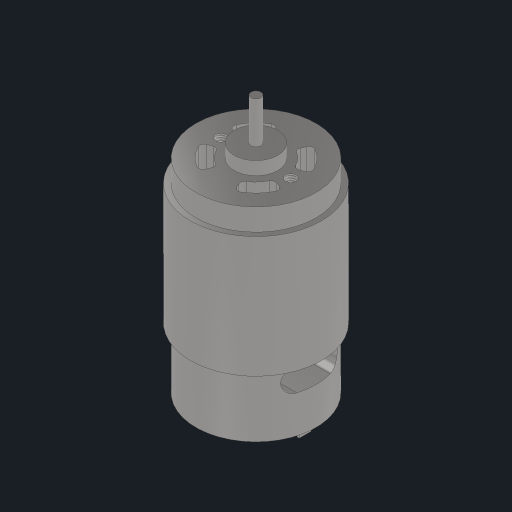
# Autodesk Inventor part: rs390
Saved by Autodesk Inventor 2023 (Build 270158000, 158)
## iProperties
Created: 2024-04-13
Part Number: rs390
Material: Steel, Mild
Document SubType Name: Modeling
Designer: szymo
Density: 3.97435 g/cm^3
Appearance: Semi-Polished
Mass: 115 g
Surface Area: 75.062 cm^2
Volume: 28.9356 cm^3
Author: szymo
Autodesk Inventor part; units mm, degrees
ref_plane "YZ Plane" through (0, 0, 0) normal (1, 0, 0) x (0, 1, 0)
sketch "Sketch1" plane through (0, 0, 0) normal (0, 1, 0) x (-1, 0, 0)
  circle A0 centre (0, 0) radius 13.75
  dimension "d0" = 27.5
  constraints: 1 centre point, 1 coincident
  measures "d0" diameter of A0
extrude "Extrusion1" add sketch "Sketch1" along normal blind 46.6
sketch "Sketch2" plane through (0, 46.6, 0) normal (0, 1, 0) x (1, 0, 0)
  circle A0 centre (0, 0) radius 13.75 projected
  circle A1 centre (0, 0) radius 5
  dimension "d3" = 10
  constraints: 1 centre point, 1 coincident
  measures "d3" diameter of A1
extrude "Extrusion2" add sketch "Sketch2" along normal blind 3 contours A1
sketch "Sketch3" plane through (0, 46.6, 0) normal (0, 1, 0) x (1, 0, 0)
  circle A0 centre (0, 0) radius 5 projected
  circle A1 centre (0, 0) radius 5 projected
  circle A2 centre (0, 0) radius 13.75 projected
  circle A3 centre (0, 0) radius 13.75 projected
  line L0 (-13.75, 0) -> (13.75, 0)
  point P0 (-8, 0)
  point P1 (8, 0)
  dimension "d6" = 16
  dimension "d7" = 5.75
  dimension "d8" = 5.75
  constraints: 2 end point, 2 point on circle, 2 point on line, 1 horizontal, 1 midpoint
  measures "d6" distance of point (-8, 0) point (8, 0)
  measures "d7" distance of L0.start point (-8, 0)
  measures "d8" distance of L0.end point (8, 0)
hole "Hole1" at (-8, 46.6, 0) at (8, 46.6, 0) direction (0, -1, 0) diameter 2.459 depth 3 thread size "M3x0.5" class "6H" standard "ISO Metric profile"
ref_plane "Work Plane1" through (0, 41.6, 0) normal (0, 1, 0) x (1, 0, 0)
sketch "Sketch4" plane through (0, 41.6, 0) normal (0, 1, 0) x (1, 0, 0)
  circle A0 centre (0, 0) radius 15
  dimension "d17" = 30
  constraints: 1 centre point, 1 coincident
  measures "d17" diameter of A0
extrude "Extrusion3" add sketch "Sketch4" against normal blind 27.7
sketch "Sketch5" plane through (0, 0, 0) normal (0, -1, 0) x (1, 0, 0)
  circle A0 centre (0, 0) radius 5
  dimension "d20" = 10
  constraints: 1 centre point, 1 coincident
  measures "d20" diameter of A0
extrude "Extrusion4" add sketch "Sketch5" along normal blind 2.7
sketch "Sketch6" plane through (0, 0, 0) normal (0, -1, 0) x (1, 0, 0)
  circle A0 centre (0, 0) radius 5 projected
  circle A1 centre (0, 0) radius 5 projected
  circle A2 centre (0, 0) radius 13.75 projected
  circle A3 centre (0, 0) radius 13.75 projected
  line L0 (13.75, 0) -> (-13.75, 0)
  line L1 (-11.25, 1.35) -> (-11.75, 1.35)
  line L2 (-11.75, 1.35) -> (-11.75, -1.35)
  line L3 (-11.75, -1.35) -> (-11.25, -1.35)
  line L4 (-11.25, -1.35) -> (-11.25, 1.35)
  line L5 (11.25, 1.35) -> (10.75, 1.35)
  line L6 (10.75, 1.35) -> (10.75, -1.35)
  line L7 (10.75, -1.35) -> (11.25, -1.35)
  line L8 (11.25, -1.35) -> (11.25, 1.35)
  dimension "d23" = 22
  dimension "d24" = 0.5
  dimension "d25" = 0.5
  dimension "d26" = 11.25
  dimension "d27" = 11.25
  dimension "d28" = 2.7
  dimension "d29" = 2.7
  dimension "d30" = 1.35
  dimension "d31" = 1.35
  constraints: 18 end point, 4 horizontal, 4 parallel, 2 perpendicular, 2 point on circle, 2 point on line
  measures "d23" distance between parallel lines of L6 L4
  measures "d24" distance of L6.end L7.end
  measures "d25" distance between parallel lines of L4 L2
  measures "d26" distance from line of A2.centre L8
  measures "d27" distance from line of A0.centre L4
  measures "d28" distance between parallel lines of L3 L1
  measures "d29" distance of L7.end L5.start
  measures "d30" distance between parallel lines of L0 L7
  measures "d31" distance between parallel lines of L0 L5
extrude "Extrusion5" add sketch "Sketch6" along normal up to surface (2.7 mm away) contours L6 L5 L8 L0 | L0 L8 L7 L6 | L4 L3 L2 L0 | L0 L2 L1 L4
sketch "Sketch7" plane through (0, 49.6, 0) normal (0, 1, 0) x (1, 0, 0)
  circle A0 centre (0, 0) radius 1.15
  dimension "d34" = 2.3
  constraints: 1 centre point, 1 coincident
  measures "d34" diameter of A0
extrude "Extrusion6" add sketch "Sketch7" along normal blind 9.5
ref_plane "Work Plane2" through (0, 50.6, 0) normal (0, 1, 0) x (1, 0, 0)
sketch "Sketch10" plane through (0, 0, 0) normal (1, 0, 0) x (0, 1, 0)
  line L0 (0, -13.75) -> (0, 13.75) projected
  line L1 (13.9, 13.75) -> (13.9, -13.75) projected
  line L2 (8.5, 3.8) -> (13.9, 3.8)
  line L3 (13.9, 3.8) -> (13.9, -3.8)
  line L4 (13.9, -3.8) -> (8.5, -3.8)
  line L5 (8.5, -3.8) -> (8.5, 3.8)
  circle A0 centre (11.2, 3.8) radius 2.7
  circle A1 centre (11.2, -3.8) radius 2.7
  line L6 (0, 0) -> (13.9, 0)
  line L7 (13.9, 13.75) -> (13.9, -13.75) projected
  line L8 (0, -13.75) -> (13.9, -13.75) projected
  point P0 (11.2, -6.5)
  point P1 (11.2, 6.5)
  dimension "d57" = 8.5
  dimension "d59" = 0
  dimension "d60" = 5.4
  dimension "d61" = 13.9
  dimension "d65" = 3.8
  dimension "d66" = 3.8
  dimension "d80" = 5.4
  dimension "d81" = 5.4
  dimension "d82" = 2.7
  dimension "d83" = 2.7
  dimension "d84" = 13
  constraints: 10 end point, 4 point on circle, 3 midpoint, 2 centre point, 2 parallel, 1 horizontal, 1 perpendicular
  measures "d57" distance between parallel lines of L0 L5
  measures "d59" distance between parallel lines of L3 L1
  measures "d60" distance between parallel lines of L5 L1
  measures "d61" distance between parallel lines of L0 L1
  measures "d65" distance from line of L6 A0.centre
  measures "d66" distance from line of L6 A1.centre
  measures "d80" diameter of A1
  measures "d81" diameter of A0
  measures "d82" distance from line of L1 A1.end
  measures "d83" distance from line of L1 A0.end
  measures "d84" distance of A0.end A1.end
extrude "Extrusion9" cut sketch "Sketch10" along normal mid plane 31.5 contours L6 L1 A1 L5 | L5 A0 L1 L6 | A1 L4 | L4 A1 | A0 L2 | L2 A0
sketch "Sketch12" plane through (0, 46.6, 0) normal (0, 1, 0) x (1, 0, 0)
  circle A0 centre (0, 0) radius 1.15 projected
  circle A1 centre (0, 0) radius 5 projected
  circle A2 centre (-8, 0) radius 1.2295 projected
  circle A3 centre (8, 0) radius 1.2295 projected
  circle A4 centre (0, 0) radius 5 projected
  circle A5 centre (0, 0) radius 13.75 projected
  circle A6 centre (0, 0) radius 13.75 projected
  line L0 (-13.75, 0) -> (13.75, 0)
  line L1 (0, 13.75) -> (0, -13.75)
  circle A7 centre (0, 0) radius 6.7705
  circle A8 centre (0, 0) radius 9.8705
  line L2 (-2.75, 6.1869) -> (-4.0091, 9.0196)
  line L3 (-6.3854, 2.2508) -> (-9.3091, 3.2814)
  line L4 (2.75, 6.1869) -> (4.0091, 9.0196)
  line L5 (6.3854, 2.2508) -> (9.3091, 3.2814)
  circle A9 centre (-8, 0) radius 1.2295 projected
  circle A10 centre (8, 0) radius 1.2295 projected
  line L6 (-2.75, -6.1869) -> (-4.0091, -9.0196)
  line L7 (-6.3854, -2.2508) -> (-9.3091, -3.2814)
  line L8 (2.75, -6.1869) -> (4.0091, -9.0196)
  line L9 (6.3854, -2.2508) -> (9.3091, -3.2814)
  point P0 (0, 6.7705)
  point P1 (0, 9.8705)
  point P2 (-8, 1.2295)
  point P3 (8, 1.2295)
  dimension "d85" = 3.1
  dimension "d86" = 5.5
  dimension "d87" = 4.0091
  dimension "d88" = 4.0091
  dimension "d89" = 1.5
  dimension "d90" = 1.5
  dimension "d91" = 1.2295
  dimension "d92" = 2.459
  dimension "d93" = 2.459
  dimension "d94" = 1.2295
  constraints: 20 end point, 14 point on circle, 8 symmetric about line, 4 line through centre, 3 midpoint, 2 centre point, 2 coincident, 2 point on line, 2 vertical alignment, 1 horizontal, 1 tangent, 1 vertical, 2 other
  measures "d85" distance of A7.start A8.start
  measures "d86" distance of L4.start L2.start
  measures "d87" distance from line of L1 L4.end
  measures "d88" horizontal distance of L2.end A8.start
  measures "d89" distance from line of point (-8, 1.23) L3
  measures "d90" distance from line of L5 point (8, 1.23)
  measures "d91" distance from line of L0 point (-8, 1.23)
  measures "d92" diameter of A2
  measures "d93" diameter of A3
  measures "d94" distance of A3.centre point (8, 1.23)
extrude "Extrusion11" cut sketch "Sketch12" against normal blind 10 contours A7 L4 A8 L5 | L9 A8 L8 A7 | A7 L3 A8 L2 | L6 A8 L7 A7
fillet "Fillet1" radius 1 16 edges at (-4.0091, 41.6, -9.0196) (-2.75, 41.6, -6.1869) (-6.3854, 41.6, -2.2508) (-9.3091, 41.6, -3.2814) (9.3091, 41.6, -3.2814) (6.3854, 41.6, -2.2508) (4.0091, 41.6, -9.0196) (9.3091, 41.6, 3.2814) (6.3854, 41.6, 2.2508) (4.0091, 41.6, 9.0196) (2.75, 41.6, 6.1869) (-4.0091, 41.6, 9.0196) (-9.3091, 41.6, 3.2814) (-6.3854, 41.6, 2.2508) (-2.75, 41.6, 6.1869) (2.75, 41.6, -6.1869)
sketch "Sketch13" plane through (0, -2.7, 0) normal (0, -1, 0) x (1, 0, 0)
  circle A0 centre (0, 0) radius 3.25
  dimension "d98" = 6.5
  constraints: 1 centre point, 1 coincident
  measures "d98" diameter of A0
extrude "Extrusion12" add sketch "Sketch13" along normal blind 1
sketch "Sketch14" plane through (0, -3.7, 0) normal (0, -1, 0) x (1, 0, 0)
  circle A0 centre (0, 0) radius 1.2
  dimension "d101" = 2.4
  constraints: 1 centre point, 1 coincident
  measures "d101" diameter of A0
extrude "Extrusion13" add sketch "Sketch14" along normal blind 1.1
equation "\"d7\" = d8"
equation "\"d26\" = d27"
equation "\"d30\" = d31"
equation "\"d65\" = d66"
equation "\"d82\" = 0.5 * d80"
equation "\"d83\" = 0.5 * d81"
equation "\"d87\" = d88"
equation "\"d91\" = 0.5 * d92"
equation "\"d94\" = 0.5 * d93"
equation "\"d41\" = d42"
body "Solid1"
